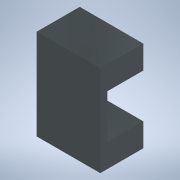
# Autodesk Inventor part: Tope_Carril
Saved by Autodesk Inventor 2022 (Build 260153000, 153)
## iProperties
Created: 2022-02-07
Part Number: Tope_Carril
Material: Generic
Document SubType Name: Modeling
Designer: katha
Density: 1 g/cm^3
Appearance: Default
Author: katha
Autodesk Inventor part; units mm, degrees
ref_plane "YZ Plane" through (0, 0, 0) normal (1, 0, 0) x (0, 1, 0)
ref_plane "XZ Plane" through (0, 0, 0) normal (0, 1, 0) x (-1, 0, 0)
ref_plane "XY Plane" through (0, 0, 0) normal (0, 0, 1) x (1, 0, 0)
sketch "Sketch1" plane through (0, 0, 0) normal (0, 0, 1) x (1, 0, 0)
  line L0 (0, 0) -> (20, 0) projected
  line L1 (20, 0) -> (20, 3.2) projected
  line L2 (0, 3.2) -> (20, 3.2) projected
  line L3 (0, 0) -> (0, 3.2) projected
  line L4 (20, -25) -> (0, -25) projected
  line L5 (0, -25) -> (0, -28.2) projected
  line L6 (20, -28.2) -> (0, -28.2) projected
  line L7 (20, -25) -> (20, -28.2) projected
  line L8 (3.2, -25) -> (3.2, 0) projected
  line L9 (0, -25) -> (0, 0) projected
  line L10 (-0.3, -0.3) -> (-0.3, 3.5)
  line L11 (-0.3, 3.5) -> (20.3, 3.5)
  line L12 (20.3, 3.5) -> (20.3, -0.3)
  line L13 (20.3, -24.7) -> (20.3, -28.5)
  line L14 (20.3, -28.5) -> (-0.3, -28.5)
  line L15 (-0.3, -28.5) -> (-0.3, -24.7)
  line L16 (3.5, -24.7) -> (3.5, -0.3)
  line L17 (-0.3, -0.3) -> (-0.3, -24.7)
  line L18 (20.3, -0.3) -> (3.5, -0.3)
  line L19 (3.5, -24.7) -> (20.3, -24.7)
  line L20 (6.5, -3.3) -> (6.5, -21.7)
  line L21 (6.5, -21.7) -> (23.3, -21.7)
  line L22 (23.3, -21.7) -> (23.3, -31.5)
  line L23 (23.3, -31.5) -> (-3.3, -31.5)
  line L24 (-3.3, -31.5) -> (-3.3, -24.7)
  line L25 (-3.3, -24.7) -> (-3.3, -0.3)
  line L26 (-3.3, -0.3) -> (-3.3, 6.5)
  line L27 (-3.3, 6.5) -> (23.3, 6.5)
  line L28 (23.3, 6.5) -> (23.3, -3.3)
  line L29 (23.3, -3.3) -> (6.5, -3.3)
  dimension "d2" = 0.3
  dimension "d3" = 0.3
  dimension "d4" = 0.3
  dimension "d5" = 24.4
  dimension "d6" = 3.8
  dimension "d7" = 3
  constraints: 40 end point, 3 equal length, 1 parallel, 13 other
  measures "d2" distance between parallel lines of L8 L16
  measures "d3" distance between parallel lines of L0 L18
  measures "d4" distance between parallel lines of L11 L2
  measures "d5" distance of L10.start L15.end
  measures "d6" distance of L10.start L10.end
  measures "d7" distance between parallel lines of L16 L20
extrude "Extrusion1" add sketch "Sketch1" against normal blind 15 contours L20 L21 L22 L23 L24 L25 L26 L27 L28 L29
sketch "Sketch4" plane through (0, 0, 0) normal (0, 0, 1) x (1, 0, 0)
  line L0 (23.3, -3.3) -> (23.3, 6.5) projected
  line L1 (23.3, 6.5) -> (-3.3, 6.5) projected
  line L2 (23.3, -3.3) -> (6.5, -3.3) projected
  line L3 (6.5, -3.3) -> (6.5, -21.7) projected
  line L4 (6.5, -21.7) -> (23.3, -21.7) projected
  line L5 (-3.3, -0.3) -> (-3.3, 6.5) projected
  line L6 (-3.3, -31.5) -> (23.3, -31.5) projected
  line L7 (23.3, -31.5) -> (23.3, -21.7) projected
  line L8 (23.3, -21.7) -> (6.5, -21.7) projected
  line L9 (23.3, 6.5) -> (23.3, -3.3) projected
  line L10 (23.3, -3.3) -> (23.3, 6.5)
  line L11 (-3.3, -31.5) -> (-3.3, 6.5) projected
  line L12 (23.3, 6.5) -> (-3.3, 6.5)
  line L13 (-3.3, 6.5) -> (-3.3, -31.5)
  line L14 (23.3, -31.5) -> (-3.3, -31.5) projected
  line L15 (-3.3, -31.5) -> (23.3, -31.5)
  line L16 (23.3, -21.7) -> (23.3, -31.5) projected
  line L17 (23.3, -31.5) -> (23.3, -21.7)
  line L18 (6.5, -3.3) -> (6.5, -21.7) projected
  line L19 (23.3, -3.3) -> (6.5, -3.3) projected
  line L20 (6.5, -3.3) -> (23.3, -3.3) projected
  line L21 (23.3, -3.3) -> (23.3, -21.7)
  point P0 (0, 0)
  constraints: 12 end point, 5 collinear, 1 perpendicular
extrude "Extrusion3" add sketch "Sketch4" along normal blind 3
sketch "Sketch5" plane through (6.5, -21.7, -15) normal (1, 0, 0) x (0, 0, -1)
  line L0 (0, 18.4) -> (0, 0) projected
  line L1 (-15, 18.4) -> (0, 18.4) projected
  line L2 (-15, 0) -> (0, 0) projected
  line L3 (-15, 0) -> (-15, 18.4) projected
  circle A0 centre (-6, 9.2) radius 2
  circle A1 centre (-6, 9.2) radius 4
  point P0 (-15, 21.7)
  dimension "d14" = 4
  dimension "d15" = 6
  dimension "d16" = 8
  dimension "d17" = 9.2
  constraints: 2 centre point, 1 coincident
  measures "d14" diameter of A0
  measures "d15" distance from line of L0 A0.centre
  measures "d16" diameter of A1
  measures "d17" distance from line of L1 A0.centre
extrude "Extrusion4" cut sketch "Sketch5" against normal blind 1 contours A1
extrude "Extrusion5" cut sketch "Sketch5" against normal blind 80 contours A0
ref_plane "Work Plane1" through (-33.2, -16.25, -125.0108) normal (0, -1, 0) x (1, 0, 0)
sketch "Sketch9" plane through (-33.2, -16.25, -125.0108) normal (0, -1, 0) x (1, 0, 0)
  line L0 (29.9, 110.0108) -> (29.9, 128.0108) projected
  circle A0 centre (15, 0) radius 2.5 projected
  line L1 (29.9, 119.0108) -> (14.9, 119.0108) construction
  line L2 (29.9, 119.0108) -> (44.9, 119.0108) construction
  line L3 (15, 0) -> (14.9, 119.0108) construction
  circle A1 centre (14.9, 119.0108) radius 2.03
  circle A2 centre (14.9, 119.0108) radius 5.03
  line L4 (14.9042, 113.9808) -> (29.9, 113.9935)
  line L5 (14.9042, 124.0408) -> (29.9, 124.0282)
  point P0 (33.2, 125.0108)
  point P1 (29.9, 113.9808)
  dimension "d27" = 15
  dimension "d28" = 180
  dimension "d29" = 4.06
  dimension "d30" = 3
  constraints: 10 end point, 3 point on line, 2 horizontal, 2 symmetric about line, 1 centre point, 1 coincident, 1 collinear, 1 midpoint, 4 other
  measures "d27" distance of L1.start L1.end
  measures "d28" angle of L1 L2
  measures "d29" diameter of A1
extrude "Extrusion7" add sketch "Sketch9" against normal blind 7.5 contours L4 A2 L5 L0 | A2
body "Solid1"
